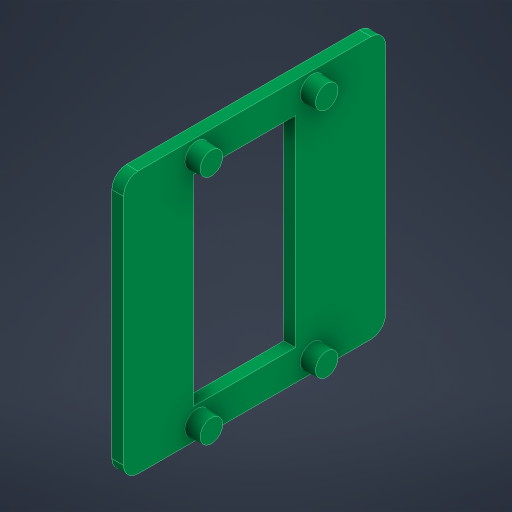
# Autodesk Inventor part: Outer Cover Side Open
Saved by Autodesk Inventor 2023.4 (Build 274418000, 418)
## iProperties
Created: 2024-07-25
Part Number: Outer Cover Side Open
Material: Generic
Document SubType Name: Modeling
Designer: xSibe
Density: 1 g/cm^3
Appearance: Plastic Dark Green
Author: xSibe
Autodesk Inventor part; units mm, degrees
ref_plane "YZ Plane" through (0, 0, 0) normal (1, 0, 0) x (0, 1, 0)
ref_plane "XZ Plane" through (0, 0, 0) normal (0, 1, 0) x (-1, 0, 0)
ref_plane "XY Plane" through (0, 0, 0) normal (0, 0, 1) x (1, 0, 0)
ref_plane "Work Plane1" through (-174.5, 24.9, 0) normal (-1, 0, 0) x (0, 0, 1)
sketch "Sketch1" plane through (-174.5, 24.9, 0) normal (-1, 0, 0) x (0, 0, 1)
  line L0 (22.875, -9.9) -> (30.375, -9.9) projected
  line L1 (30.375, -9.9) -> (30.375, -39.9) projected
  line L2 (30.375, -39.9) -> (22.875, -39.9) projected
  line L3 (22.875, -39.9) -> (22.875, -9.9) projected
  line L4 (0.025, -47.8) -> (0.025, -2) projected
  line L5 (42.1, -47.8) -> (0.025, -47.8) projected
  line L6 (42.1, -47.8) -> (42.1, -2) projected
  line L7 (0.025, -2) -> (42.1, -2) projected
  circle A0 centre (34.8, -44.8) radius 2.0625 projected
  circle A1 centre (34.8, -5) radius 2.0625 projected
  circle A2 centre (15, -44.8) radius 2.0625 projected
  circle A3 centre (15, -5) radius 2.0625 projected
  spline S0 degree 2 poles (48.6069, -31.7514) (48.3745, -32.0925) (47.6578, -32.478) (47.1486, -32.478) knots 0 0 0 1 2 2 2 projected
  spline S1 degree 2 poles (47.1486, -32.478) (46.7531, -32.478) (46.0413, -32.1963) (45.7941, -31.9442) knots 0 0 0 1 2 2 2 projected
  spline S2 degree 2 poles (45.7941, -31.9442) (45.4827, -31.6278) (45.1614, -30.7726) (45.1614, -30.1201) knots 0 0 0 1 2 2 2 projected
  line L8 (45.1614, -30.1201) -> (45.1614, -29.433) projected
  line L9 (45.1614, -29.433) -> (42.8875, -29.433) projected
  line L10 (42.8875, -29.433) -> (42.8875, -28.6223) projected
  line L11 (42.8875, -28.6223) -> (48.9875, -28.6223) projected
  line L12 (48.9875, -28.6223) -> (48.9875, -30.1547) projected
  spline S3 degree 2 poles (48.9875, -30.1547) (48.9875, -30.6985) (48.8095, -31.4597) (48.6069, -31.7514) knots 0 0 0 1 2 2 2 projected
  spline S4 degree 2 poles (49.116, -25.0335) (49.116, -25.6563) (48.681, -26.6549) (48.2905, -27.0009) knots 0 0 0 1 2 2 2 projected
  spline S5 degree 2 poles (48.2905, -27.0009) (47.8852, -27.3469) (46.6988, -27.7325) (45.9375, -27.7325) knots 0 0 0 1 2 2 2 projected
  spline S6 degree 2 poles (45.9375, -27.7325) (45.196, -27.7325) (43.9948, -27.3568) (43.5894, -27.0009) knots 0 0 0 1 2 2 2 projected
  spline S7 degree 2 poles (43.5894, -27.0009) (43.1643, -26.6252) (42.759, -25.6316) (42.759, -25.0335) knots 0 0 0 1 2 2 2 projected
  spline S8 degree 2 poles (42.759, -25.0335) (42.759, -24.4156) (43.1792, -23.4269) (43.5894, -23.066) knots 0 0 0 1 2 2 2 projected
  spline S9 degree 2 poles (43.5894, -23.066) (43.9948, -22.7151) (45.1861, -22.3394) (45.9375, -22.3394) knots 0 0 0 1 2 2 2 projected
  spline S10 degree 2 poles (45.9375, -22.3394) (46.7037, -22.3394) (47.8703, -22.72) (48.2905, -23.071) knots 0 0 0 1 2 2 2 projected
  spline S11 degree 2 poles (48.2905, -23.071) (48.6958, -23.4269) (49.116, -24.4205) (49.116, -25.0335) knots 0 0 0 1 2 2 2 projected
  line L13 (42.8875, -20.021) -> (42.8875, -19.2103) projected
  line L14 (42.8875, -19.2103) -> (48.2658, -19.2103) projected
  line L15 (48.2658, -19.2103) -> (48.2658, -17.1638) projected
  line L16 (48.2658, -17.1638) -> (48.9875, -17.1638) projected
  line L17 (48.9875, -17.1638) -> (48.9875, -22.0675) projected
  line L18 (48.9875, -22.0675) -> (48.2658, -22.0675) projected
  line L19 (48.2658, -22.0675) -> (48.2658, -20.021) projected
  line L20 (48.2658, -20.021) -> (42.8875, -20.021) projected
  line L21 (49.775, -2) -> (49.775, -47.8) projected
  line L22 (42.1, -2) -> (49.775, -2) projected
  line L23 (42.1, -2) -> (42.1, -47.8) projected
  line L24 (49.775, -47.8) -> (42.1, -47.8) projected
  line L25 (49.775, -2) -> (0.025, -2)
  line L26 (0.025, -2) -> (0.025, -47.8)
  line L27 (0.025, -47.8) -> (49.775, -47.8)
  line L28 (49.775, -47.8) -> (49.775, -2)
  line L29 (24.9, -2) -> (24.9, -47.8)
  line L30 (4.9, -2.4) -> (44.9, -2.4)
  line L31 (47.4, -4.9) -> (47.4, -44.9)
  line L32 (44.9, -47.4) -> (4.9, -47.4)
  line L33 (2.4, -44.9) -> (2.4, -4.9)
  line L34 (2.4, -2.4) -> (47.4, -47.4) construction
  line L35 (47.4, -2.4) -> (2.4, -47.4) construction
  arc A4 (47.4, -4.9) -> (44.9, -2.4) centre (44.9, -4.9) ccw
  arc A5 (44.9, -47.4) -> (47.4, -44.9) centre (44.9, -44.9) ccw
  arc A6 (2.4, -44.9) -> (4.9, -47.4) centre (4.9, -44.9) ccw
  arc A7 (4.9, -2.4) -> (2.4, -4.9) centre (4.9, -4.9) ccw
  line L36 (35.375, -44.9) -> (35.375, -4.9)
  line L37 (35.375, -4.9) -> (17.875, -4.9)
  line L38 (17.875, -4.9) -> (17.875, -44.9)
  line L39 (17.875, -44.9) -> (35.375, -44.9)
  line L40 (2.4, -42.15) -> (47.4, -42.15)
  line L41 (47.4, -42.15) -> (47.4, -7.65)
  line L42 (47.4, -7.65) -> (2.4, -7.65)
  line L43 (2.4, -7.65) -> (2.4, -42.15)
  line L44 (2.4, -42.15) -> (47.4, -7.65) construction
  line L45 (47.4, -42.15) -> (2.4, -7.65) construction
  point P0 (0, -24.9)
  point P1 (24.9, -24.9)
  point P2 (17.875, -42.15)
  point P3 (17.875, -7.65)
  point P4 (35.375, -7.65)
  point P5 (35.375, -42.15)
  dimension "d0" = 45
  dimension "d1" = 45
  dimension "d2" = 2.5
  dimension "d3" = 5
  dimension "d4" = 34.5
  constraints: 42 end point, 9 point on line, 8 point on circle, 8 tangent, 7 midpoint, 6 parallel, 4 centre point, 3 equal radius, 3 horizontal, 3 perpendicular, 3 other
  measures "d0" distance of L34.end L35.end
  measures "d1" distance of L35.start L34.end
  measures "d2" radius of A4
  measures "d3" distance between parallel lines of L1 L36
  measures "d4" distance of L41.end L40.end
extrude "Extrusion1" add sketch "Sketch1" along normal blind 2 contours L42 L38 L37 L29 | L29 L37 A1 L36 L42 | L37 L38 L42 L33 A7 L30 L29 | L29 L30 L6 L42 L36 A1 L37 | L42 L6 L40 L36 | L38 L40 L33 L42 | L40 L36 A0 L39 L29 | L29 L39 L38 L40 | L37 L36 A1 | A1 L36 L37 | L40 L6 L32 L29 L39 A0 L36 | L42 L31 L14 L13 L20 S10 S9 S8 S7 S6 S5 L11 L10 L9 L8 S2 S1 S0 L40 L6 | L6 L30 A4 L31 L42 | L38 L39 L29 L32 A6 L33 L40 | L36 L39 A0 | A0 L39 L36 | L40 L31 A5 L32 L6 | L31 L20 L13 L14 | S0 S1 S2 L8 L9 L10 L11 L31 | L31 S5 S6 S7 S8 S9 S10 | A2 | A3
sketch "Sketch2" plane through (-174.5, 24.9, 0) normal (1, 0, 0) x (0, 0, -1)
  line L0 (-22.875, -9.9) -> (-30.375, -9.9) projected
  line L1 (-30.375, -9.9) -> (-30.375, -39.9) projected
  line L2 (-30.375, -39.9) -> (-22.875, -39.9) projected
  line L3 (-22.875, -39.9) -> (-22.875, -9.9) projected
  line L4 (-0.025, -47.8) -> (-0.025, -2) projected
  line L5 (-42.1, -47.8) -> (-0.025, -47.8) projected
  line L6 (-42.1, -47.8) -> (-42.1, -2) projected
  line L7 (-0.025, -2) -> (-42.1, -2) projected
  circle A0 centre (-34.8, -44.8) radius 2.0625 projected
  circle A1 centre (-34.8, -5) radius 2.0625 projected
  circle A2 centre (-15, -44.8) radius 2.0625 projected
  circle A3 centre (-15, -5) radius 2.0625 projected
  point P0 (0, -24.9)
ref_plane "Work Plane2" through (-172, 17.8375, 32.7375) normal (-1, 0, 0) x (0, 0, 1)
extrude "Extrusion2" add sketch "Sketch2" along normal up to surface (2.5 mm away) contours A0 | A1 | A2 | A3
chamfer "Chamfer1" distance 0.125 distance2 2.5 1 edges at (-172, 19.9, 36.8625) measured on face at (-172, 19.9, 36.3625)
chamfer "Chamfer2" distance 0.125 distance2 2.5 1 edges at (-172, 19.9, 17.0625) measured on face at (-172, 19.9, 16.5625)
chamfer "Chamfer3" distance 0.125 distance2 2.5 1 edges at (-172, -19.9, 36.8625) measured on face at (-172, -19.9, 36.3625)
chamfer "Chamfer4" distance 0.125 distance2 2.5 1 edges at (-172, -19.9, 17.0625) measured on face at (-172, -19.9, 16.5625)
body "Solid1"
